# Autodesk Inventor part: NanoCaseBottom
Saved by Autodesk Inventor 2014 SP1 (Build 180222100, 222)
## iProperties
Created: 2017-05-21
Part Number: NanoCaseBottom
Material: ABS Plastic
Document SubType Name: Modeling
Designer: danielsikar
Density: 1.06 g/cm^3
Appearance: Smooth - White
Author: danielsikar
Autodesk Inventor part; units mm, degrees
ref_plane "YZ Plane" through (0, 0, 0) normal (1, 0, 0) x (0, 1, 0)
ref_plane "XZ Plane" through (0, 0, 0) normal (0, 1, 0) x (-1, 0, 0)
ref_plane "Work Plane1" through (25.9939, 2.4534, 2.2732) normal (0, 0, -1) x (-1, 0, 0)
sketch "Sketch1" plane through (25.9939, 2.4534, 2.2732) normal (0, 0, -1) x (-1, 0, 0)
  line L0 (21.65, -9.18) -> (-21.65, -9.18) projected
  line L1 (21.65, 9.18) -> (21.65, -9.18) projected
  line L2 (-21.65, 9.18) -> (21.65, 9.18) projected
  line L3 (-21.65, -9.18) -> (-21.65, 9.18) projected
  line L4 (24.65, 12.18) -> (24.65, -12.18)
  line L5 (24.65, -12.18) -> (-23.17, -12.18)
  line L6 (-23.17, 12.18) -> (24.65, 12.18)
  line L7 (-23.17, 3.98) -> (-23.17, -3.6) projected
  line L8 (-23.17, 12.18) -> (-23.17, -12.18)
  point P0 (25.9939, -2.4534)
  dimension "d0" = 3
  constraints: 8 end point, 1 perpendicular
  measures "d0" distance between parallel lines of L6 L2
extrude "Extrusion1" add sketch "Sketch1" along normal blind 2 contours L0 L3 L2 L1 | L4 L5 L8 L7 L6
sketch "Sketch2" plane through (25.9939, 2.4534, 2.2732) normal (0, 0, 1) x (1, 0, 0)
  line L0 (-24.65, 12.18) -> (-24.65, -12.18) projected
  line L1 (-24.65, -12.18) -> (23.17, -12.18) projected
  line L2 (21.65, 9.18) -> (-21.65, 9.18) projected
  line L3 (-21.65, 9.18) -> (-21.65, -9.18) projected
  line L4 (-21.65, -9.18) -> (21.65, -9.18) projected
  line L5 (21.65, -10.18) -> (-22.65, -10.18)
  line L6 (-22.65, -10.18) -> (-22.65, 10.18)
  line L7 (-22.65, 10.18) -> (21.65, 10.18)
  line L8 (21.65, 10.18) -> (21.65, -10.18)
  line L9 (-24.65, 12.18) -> (23.17, 12.18)
  line L10 (23.17, 12.18) -> (23.17, -12.18)
  line L11 (23.17, -12.18) -> (-24.65, -12.18)
  line L12 (-24.65, -12.18) -> (-24.65, 12.18)
  point P0 (-25.9939, -2.4534)
  dimension "d3" = 1
  constraints: 16 end point, 2 parallel, 2 perpendicular, 1 horizontal, 2 other
  measures "d3" distance between parallel lines of L5 L4
extrude "Extrusion2" add sketch "Sketch2" along normal blind 8
sketch "Sketch4" plane through (25.9939, 2.4534, 10.2732) normal (0, 0, 1) x (1, 0, 0)
  line L0 (21.65, 10.18) -> (21.65, -10.18) projected
  line L1 (23.17, 3.98) -> (13.97, 3.98) construction
  line L2 (13.97, -3.6) -> (23.17, -3.6) construction
  line L3 (21.65, 3.98) -> (23.17, 3.98)
  line L4 (23.17, 3.98) -> (23.17, -3.6)
  line L5 (23.17, -3.6) -> (21.65, -3.6)
  line L6 (21.65, -3.6) -> (21.65, 3.98)
  point P0 (-25.9939, -2.4534)
  constraints: 8 end point, 2 parallel, 2 point on line, 1 horizontal, 1 perpendicular
ref_plane "Work Plane2" through (4.3439, -6.7266, 5.9732) normal (0, 0, 1) x (1, 0, 0)
extrude "Extrusion4" cut sketch "Sketch4" against normal up to surface (4.3 mm away)
sketch "Sketch5" plane through (47.6439, -1.1466, 10.2732) normal (0, 1, 0) x (1, 0, 0)
  line L0 (1.52, 4.3) -> (0, 4.3) projected
  line L1 (0, 0) -> (0, 4.3) projected
  line L2 (1.52, 0) -> (0, 0) projected
  line L3 (1.52, 4.3) -> (1.52, 0) projected
  point P0 (-47.6439, 10.2732)
extrude "Extrusion5" cut sketch "Sketch5" against normal blind 0.3
sketch "Sketch6" plane through (47.6439, 6.4334, 10.2732) normal (0, -1, 0) x (1, 0, 0)
  line L0 (0, -4.3) -> (1.52, -4.3) projected
  line L1 (1.52, 0) -> (1.52, -4.3) projected
  line L2 (0, 0) -> (1.52, 0) projected
  line L3 (0, -4.3) -> (0, 0) projected
  point P0 (-47.6439, -10.2732)
extrude "Extrusion6" cut sketch "Sketch6" against normal blind 0.3
sketch "Sketch7" plane through (47.6439, 6.7334, 10.2732) normal (0, -1, 0) x (1, 0, 0)
  line L0 (1.52, 0) -> (1.52, -4.3) projected
  line L1 (0, 0) -> (1.52, 0) projected
  line L2 (0, -4.3) -> (0, 0) projected
  line L3 (0, 0) -> (1.52, 0)
  line L4 (1.52, 0) -> (1.52, -2)
  line L5 (1.52, -2) -> (0, -2)
  line L6 (0, -2) -> (0, 0)
  point P0 (-47.6439, -10.2732)
  dimension "d14" = 2
  dimension "d15" = 0
  constraints: 8 end point, 2 parallel, 2 point on line, 1 horizontal, 1 perpendicular
  measures "d14" distance of L3.end L4.end
  measures "d15" distance between parallel lines of L1 L3
extrude "Extrusion7" cut sketch "Sketch7" against normal blind 4
sketch "Sketch8" plane through (25.9939, 2.4534, 2.2732) normal (0, 0, 1) x (1, 0, 0)
  line L0 (-22.65, 10.18) -> (-20.15, 10.18)
  line L1 (-20.15, 10.18) -> (-20.15, 7.68)
  line L2 (-20.15, 7.68) -> (-22.65, 7.68)
  line L3 (-22.65, 7.68) -> (-22.65, 10.18)
  line L4 (21.65, 10.18) -> (19.15, 10.18)
  line L5 (19.15, 10.18) -> (19.15, 7.68)
  line L6 (19.15, 7.68) -> (21.65, 7.68)
  line L7 (21.65, 7.68) -> (21.65, 10.18)
  line L8 (-22.65, -10.18) -> (-20.15, -10.18)
  line L9 (-20.15, -10.18) -> (-20.15, -7.68)
  line L10 (-20.15, -7.68) -> (-22.65, -7.68)
  line L11 (-22.65, -7.68) -> (-22.65, -10.18)
  line L12 (21.65, -10.18) -> (19.15, -10.18)
  line L13 (19.15, -10.18) -> (19.15, -7.68)
  line L14 (19.15, -7.68) -> (21.65, -7.68)
  line L15 (21.65, -7.68) -> (21.65, -10.18)
  point P0 (-25.9939, -2.4534)
  dimension "d18" = 2.5
  dimension "d19" = 2.5
  dimension "d20" = 2.5
  dimension "d21" = 2.5
  dimension "d22" = 2.5
  dimension "d23" = 2.5
  constraints: 32 end point, 8 parallel, 4 horizontal, 4 perpendicular
  measures "d18" distance of L1.end L2.end
  measures "d19" distance of L0.end L1.end
  measures "d20" distance of L6.end L5.end
  measures "d21" distance of L9.end L8.end
  measures "d22" distance of L13.end L14.end
  measures "d23" distance of L12.end L13.end
extrude "Extrusion8" add sketch "Sketch8" along normal blind 2
fillet "Fillet1" radius 2 4 edges at (49.1639, 14.6334, 5.2732) (49.1639, -9.7266, 5.2732) (1.3439, 14.6334, 5.2732) (1.3439, -9.7266, 5.2732)
body "Solid1"
